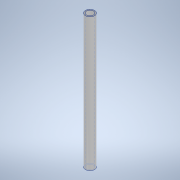
# Autodesk Inventor part: ロボット回転_ベアリングシャフト横
Saved by Autodesk Inventor 2020.3 (Build 243373000, 373)
## iProperties
Created: 2020-07-05
Part Number: ロボット回転_ベアリングシャフト横
Material: アルミニウム 6061
Document SubType Name: Modeling
Designer: totot
Density: 2.7 g/cm^3
Appearance: アルミニウム - フラット
Mass: 0.616027 g
Surface Area: 9.23628 cm^2
Volume: 0.228158 cm^3
Author: totot
Autodesk Inventor part; units mm, degrees
ref_plane "YZ Plane" through (0, 0, 0) normal (1, 0, 0) x (0, 1, 0)
ref_plane "XZ Plane" through (0, 0, 0) normal (0, 1, 0) x (-1, 0, 0)
ref_plane "XY Plane" through (0, 0, 0) normal (0, 0, 1) x (1, 0, 0)
sketch "スケッチ1" plane through (0, 0, 0) normal (0, 1, 0) x (-1, 0, 0)
  circle A0 centre (0, 0) radius 2
  dimension "d0" = 4
  constraints: 1 centre point, 1 coincident
  measures "d0" diameter of A0
extrude "押し出し1" add sketch "スケッチ1" along normal blind 50.5
sketch "スケッチ2" plane through (0, 50.5, 0) normal (0, 1, 0) x (1, 0, 0)
  point P0 (0, 0)
  point P1 (0, 0)
  constraints: 1 coincident
hole "穴1" at (0, 50.5, 0) direction (0, -1, 0) diameter 3 end through all
